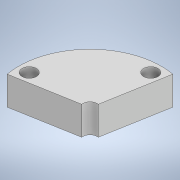
# Autodesk Inventor part: bell_crank_small_v1
Saved by Autodesk Inventor 2022 (Build 260153000, 153)
## iProperties
Created: 2022-05-22
Part Number: bell_crank_small_v1
Material: Generic
Document SubType Name: Modeling
Designer: kylem
Density: 1 g/cm^3
Appearance: Default
Author: kylem
Autodesk Inventor part; units mm, degrees
ref_plane "YZ Plane" through (0, 0, 0) normal (1, 0, 0) x (0, 1, 0)
ref_plane "XZ Plane" through (0, 0, 0) normal (0, 1, 0) x (-1, 0, 0)
ref_plane "XY Plane" through (0, 0, 0) normal (0, 0, 1) x (1, 0, 0)
sketch "Sketch1" plane through (0, 0, 0) normal (0, 1, 0) x (-1, 0, 0)
  circle A0 centre (0, 0) radius 10
  line L0 (0, 0) -> (9.8481, 1.7365)
  line L1 (0, 0) -> (10, 0) construction
  line L2 (0, 0) -> (-1.7365, -9.8481)
  line L3 (0, 0) -> (10, 0) construction
  line L4 (10, 0) -> (8.5, 0)
  circle A1 centre (8.5, 0) radius 1
  line L5 (0, -10) -> (0, -8.5)
  circle A2 centre (0, -8.5) radius 1
  dimension "d0" = 20
  dimension "d1" = 10
  dimension "d2" = 100
  dimension "d3" = 1.5
  dimension "d4" = 2
  dimension "d5" = 1.5
  dimension "d6" = 2
  constraints: 12 end point, 3 centre point, 3 coincident, 3 point on circle, 2 equal length, 2 horizontal, 1 point on line, 1 vertical
  measures "d0" diameter of A0
  measures "d1" angle of L1 L0
  measures "d2" angle of L2 L3
  measures "d3" distance of L3.end L4.end
  measures "d4" diameter of A1
  measures "d5" distance of L5.start L5.end
  measures "d6" diameter of A2
extrude "Extrusion1" add sketch "Sketch1" along normal blind 4 contours A0 L2 L0 picked at (2.2606, -5.1604)
sketch "Sketch2" plane through (0, 4, 0) normal (0, 1, 0) x (1, 0, 0)
  line L0 (0, 0) -> (1.7365, 9.8481) projected
  circle A0 centre (0, 0) radius 1
  dimension "d9" = 2
  constraints: 1 centre point, 1 coincident
  measures "d9" diameter of A0
extrude "Extrusion2" cut sketch "Sketch2" against normal blind 4
body "Solid1"
